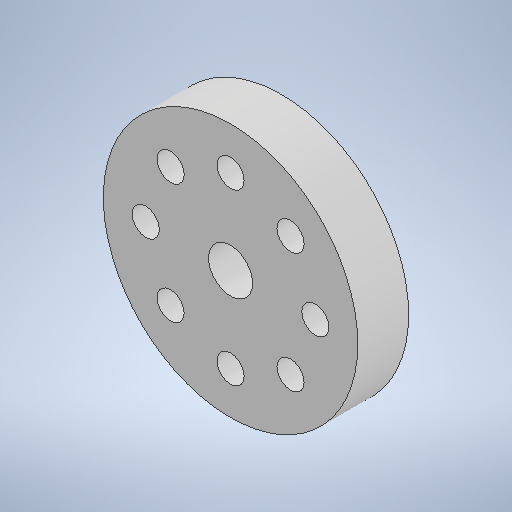
# Autodesk Inventor part: dentatu
Saved by Autodesk Inventor 2025.1 (Build 291241000, 241)
## iProperties
Created: 2024-08-31
Part Number: dentatu
Material: 一般
Document SubType Name: Modeling
Designer: right
Density: 1 g/cm^3
Appearance: 既定
Author: right
Autodesk Inventor part; units mm, degrees
ref_plane "YZ Plane" through (0, 0, 0) normal (1, 0, 0) x (0, 1, 0)
ref_plane "XZ Plane" through (0, 0, 0) normal (0, 1, 0) x (-1, 0, 0)
ref_plane "XY Plane" through (0, 0, 0) normal (0, 0, 1) x (1, 0, 0)
sketch "スケッチ1" plane through (0, 0, 0) normal (0, 0, 1) x (1, 0, 0)
  circle A0 centre (0, 0) radius 7.5
  circle A1 centre (0, 0) radius 5 construction
  circle A2 centre (0, 5) radius 0.8
  circle A3 centre (-3.5355, 3.5355) radius 0.8
  circle A4 centre (-5, 0) radius 0.8
  circle A5 centre (-3.5355, -3.5355) radius 0.8
  circle A6 centre (0, -5) radius 0.8
  circle A7 centre (3.5355, -3.5355) radius 0.8
  circle A8 centre (5, 0) radius 0.8
  circle A9 centre (3.5355, 3.5355) radius 0.8
  circle A10 centre (0, 0) radius 1.3
  dimension "d1" = 10
  dimension "d0" = 15
  dimension "d2" = 1.6
  dimension "d5" = 360
  dimension "d7" = 2.6
  constraints: 10 centre point, 3 coincident, 2 vertical alignment, 19 other
  measures "d0" diameter of A0
  measures "d2" diameter of A2
  measures "d7" diameter of A10
extrude "押し出し1" add sketch "スケッチ1" along normal blind 3
